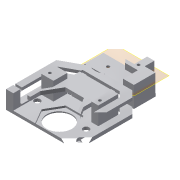
# Autodesk Inventor part: 06_Case_Upper_v1
Saved by Autodesk Inventor 2016 (Build 200138000, 138)
## iProperties
Created: 2017-11-17
Part Number: 06_Case_Upper_v1
Material: Generisch
Document SubType Name: Modeling
Designer: diederichbenedict
Density: 1 g/cm^3
Appearance: Weiß
Author: diederichbenedict
Autodesk Inventor part; units mm, degrees
ref_plane "YZ Plane" through (0, 0, 0) normal (1, 0, 0) x (0, 1, 0)
ref_plane "XZ Plane" through (0, 0, 0) normal (0, 1, 0) x (-1, 0, 0)
ref_plane "XY Plane" through (0, 0, 0) normal (0, 0, 1) x (1, 0, 0)
ref_plane "Arbeitsebene1" through (-53, 10.5, 0) normal (0, 0, 1) x (1, 0, 0)
sketch "Skizze1" plane through (-53, 10.5, 0) normal (0, 0, 1) x (1, 0, 0)
  circle A0 centre (53, -7.5) radius 1.75 construction
  line L0 (49, 8.5) -> (49, -12.5) construction
  line L1 (49, -12.5) -> (57, -12.5) construction
  line L2 (57, -12.5) -> (57, 8.5) construction
  line L3 (57, 8.5) -> (49, 8.5) construction
  arc A1 (1.4361, -8.5) -> (-1.4361, -8.5) centre (0, -7.5) ccw construction
  line L4 (1.4361, -8.5) -> (4, -8.5) construction
  line L5 (4, -8.5) -> (4, 8.5) construction
  line L6 (4, 8.5) -> (-4, 8.5) construction
  line L7 (-4, 8.5) -> (-4, -8.5) construction
  line L8 (-4, -8.5) -> (-1.4361, -8.5) construction
  line L9 (74, -106.5) -> (69, -111.5) construction
  line L10 (74, -66.5) -> (74, -106.5) construction
  line L11 (64, -66.5) -> (74, -66.5) construction
  line L12 (64, -70.0238) -> (64, -66.5) construction
  line L13 (71.5194, -70.0238) -> (64, -70.0238) construction
  line L14 (71.5194, -74.0238) -> (71.5194, -70.0238) construction
  line L15 (64, -74.0238) -> (71.5194, -74.0238) construction
  line L16 (64, -111.5) -> (64, -74.0238) construction
  line L17 (69, -111.5) -> (64, -111.5) construction
  circle A2 centre (69, -77.2738) radius 1.75 construction
  circle A3 centre (1, -79.0238) radius 1.75 construction
  line L18 (1, -74.0238) -> (6, -82.684) construction
  line L19 (-1, -74.0238) -> (1, -74.0238) construction
  line L20 (-1, -70.0238) -> (-1, -74.0238) construction
  line L21 (0.3943, -66.5) -> (-1, -70.0238) construction
  line L22 (-4, -66.5) -> (0.3943, -66.5) construction
  line L23 (-4, -106.5) -> (-4, -66.5) construction
  line L24 (1, -111.5) -> (-4, -106.5) construction
  line L25 (6, -111.5) -> (1, -111.5) construction
  line L26 (6, -82.684) -> (6, -111.5) construction
  line L27 (-4, -111.5) -> (-4, 8.5) construction
  line L28 (-4, 8.5) -> (4, 8.5) construction
  line L29 (6, 8.5) -> (4, 8.5) construction
  line L30 (74, -66.5) -> (6, -66.5) construction
  line L31 (74, -111.5) -> (74, -66.5) construction
  circle A4 centre (38.7332, -103.6375) radius 17.5 construction
  circle A5 centre (13, 28.5) radius 1 construction
  circle A6 centre (43, -3.5) radius 1 construction
  circle A7 centre (13, -3.5) radius 1 construction
  circle A8 centre (43, 28.5) radius 1 construction
  circle A9 centre (28, 12.5) radius 18.75 construction
  line L32 (48, -3.5) -> (48, 28.5) construction
  arc A10 (43, -8.5) -> (48, -3.5) centre (43, -3.5) ccw construction
  line L33 (13, -8.5) -> (43, -8.5) construction
  arc A11 (8, -3.5) -> (13, -8.5) centre (13, -3.5) ccw construction
  line L34 (8, 28.5) -> (8, -3.5) construction
  arc A12 (13, 33.5) -> (8, 28.5) centre (13, 28.5) ccw construction
  line L35 (43, 33.5) -> (13, 33.5) construction
  arc A13 (48, 28.5) -> (43, 33.5) centre (43, 28.5) ccw construction
  line L36 (74, -111.5) -> (74, -125) construction
  line L37 (74, -125) -> (-4, -125) construction
  line L38 (-4, -125) -> (-4, -111.5) construction
  circle A14 centre (38.7332, -103.6375) radius 17.5 construction
  line L39 (57, 8.5) -> (49, 8.5) construction
  line L40 (49, 8.5) -> (49, -9.5) construction
  line L41 (49, -12.5) -> (57, -12.5) construction
  line L42 (57, -12.5) -> (57, 8.5) construction
  line L43 (6, -9.5) -> (49, -9.5) construction
  line L44 (57, -12.5) -> (49, -12.5) construction
  line L45 (6, -14.5) -> (57, -14.5) construction
  line L46 (57, -14.5) -> (57, -12.5) construction
  line L47 (6, -66.5) -> (6, -14.5) construction
  line L48 (6, -9.5) -> (6, 8.5) construction
  line L49 (49, -12.5) -> (48, -12.5) construction
  line L50 (-4, 8.5) -> (6, 8.5)
  line L51 (6, 8.5) -> (6, -9.5)
  line L52 (6, -9.5) -> (49, -9.5)
  line L53 (49, -9.5) -> (49, 8.5)
  line L54 (57, 8.5) -> (49, 8.5)
  line L55 (57, 8.5) -> (57, -14.5)
  line L56 (57, -14.5) -> (6, -14.5)
  line L57 (6, -14.5) -> (6, -66.5)
  line L58 (6, -66.5) -> (74, -66.5)
  line L59 (74, -66.5) -> (74, -125)
  line L60 (74, -125) -> (-4, -125)
  line L61 (-4, -125) -> (-4, 8.5)
  circle A15 centre (38.7332, -103.6375) radius 17.5
  circle A16 centre (1, -96.5) radius 4.25
  circle A17 centre (69, -96.5) radius 4.25
  circle A18 centre (0, 3.5) radius 3.5
  circle A19 centre (53, 3.5) radius 3.5
  line L62 (57, 8.5) -> (59, 8.5)
  line L63 (59, 8.5) -> (59, -14.5)
  line L64 (59, -14.5) -> (57, -14.5)
  line L65 (57, -14.5) -> (57, 8.5)
  line L66 (6, -14.5) -> (13, -14.5)
  line L67 (13, -14.5) -> (13, -66.5)
  line L68 (13, -66.5) -> (6, -66.5)
  line L69 (6, -66.5) -> (6, -14.5)
  line L70 (74, -106.5) -> (69, -111.5) projected
  line L71 (74, -66.5) -> (74, -106.5) projected
  line L72 (64, -70.0238) -> (64, -66.5) projected
  line L73 (71.5194, -70.0238) -> (64, -70.0238) projected
  line L74 (71.5194, -74.0238) -> (71.5194, -70.0238) projected
  line L75 (64, -74.0238) -> (71.5194, -74.0238) projected
  line L76 (64, -111.5) -> (64, -74.0238) projected
  line L77 (69, -111.5) -> (64, -111.5) projected
  arc A20 (1.4361, -8.5) -> (1, -8.9361) centre (0, -7.5) ccw projected
  line L78 (1.4361, -8.5) -> (4, -8.5) projected
  line L79 (4, -8.5) -> (4, 8.5) projected
  line L80 (4, 8.5) -> (-4, 8.5) projected
  line L81 (-4, 8.5) -> (-4, -19.0851) projected
  line L82 (49, 8.5) -> (49, -12.5) projected
  line L83 (57, 8.5) -> (49, 8.5) projected
  line L84 (59, -14.5) -> (74, -14.5)
  line L85 (74, -14.5) -> (74, -4.5)
  line L86 (74, -4.5) -> (59, -4.5)
  line L87 (59, -4.5) -> (59, -14.5)
  line L88 (74, -14.5) -> (59, -14.5)
  line L89 (59, -14.5) -> (59, -35)
  line L90 (59, -35) -> (74, -35)
  line L91 (74, -35) -> (74, -14.5)
  line L92 (-4, -19.0851) -> (1, -19.0851) projected
  line L93 (1, -19.0851) -> (1, -8.9361) projected
  circle A21 centre (1, -96.5) radius 3.75 projected
  circle A22 centre (69, -96.5) radius 3.75 projected
  circle A23 centre (0, 3.5) radius 3 projected
  circle A24 centre (53, 3.5) radius 3 projected
  point P0 (53, -10.5)
  dimension "d1" = 2
  dimension "d2" = 8.5
  dimension "d3" = 8.5
  dimension "d4" = 7
  dimension "d5" = 7
  constraints: 95 end point, 21 perpendicular, 13 parallel, 8 horizontal, 8 point on line, 6 centre point, 3 vertical, 2 coincident, 1 collinear, 1 concentric
  measures "d1" distance between parallel lines of L45 L44
  measures "d2" diameter of A16
  measures "d3" diameter of A17
  measures "d4" diameter of A18
  measures "d5" diameter of A19
extrude "Extrusion1" add sketch "Skizze1" along normal blind 4 contours L50 L79 L78 A20 L93 L92 L61 | L50 L51 L52 L53 L54 L55 L56 L57 L58 L72 L73 L74 L75 L76 L77 L70 L59 L60 L61 L92 L93 A20 L78 L79 | L70 L77 L76 L75 L74 L73 L72 L58 L59 | L62 L63 L64 L55 | L58 L57 L56 L67 | L63 L86 L85 L84 | L84 L91 L90 L89
sketch "Skizze2" plane through (-53, 10.5, 4) normal (0, 0, 1) x (1, 0, 0)
  circle A0 centre (38.7332, -103.6375) radius 18 construction
  line L0 (50.5689, -124.1375) -> (62.4046, -103.6375) construction
  line L1 (62.4046, -103.6375) -> (50.5689, -83.1375) construction
  line L2 (50.5689, -83.1375) -> (26.8975, -83.1375) construction
  line L3 (26.8975, -83.1375) -> (15.0619, -103.6375) construction
  line L4 (15.0619, -103.6375) -> (26.8975, -124.1375) construction
  line L5 (26.8975, -124.1375) -> (50.5689, -124.1375) construction
  line L6 (51.0601, -82.2867) -> (63.387, -103.6375)
  line L7 (63.387, -103.6375) -> (51.0601, -124.9883)
  line L8 (51.0601, -124.9883) -> (26.4063, -124.9883)
  line L9 (26.4063, -124.9883) -> (14.0795, -103.6375)
  line L10 (14.0795, -103.6375) -> (26.4063, -82.2867)
  line L11 (26.4063, -82.2867) -> (51.0601, -82.2867)
  point P0 (53, -10.5)
  dimension "d8" = 0.8508
  constraints: 12 end point, 5 other
  measures "d8" distance between parallel lines of L1 L6
extrude "Extrusion2" cut sketch "Skizze2" against normal blind 2.5
sketch "Skizze4" plane through (-53, 10.5, 0) normal (0, 0, -1) x (-1, 0, 0)
  circle A0 centre (-38.7332, -103.6375) radius 17.5 projected
  circle A1 centre (-69, -96.5) radius 4.25 projected
  circle A2 centre (-1, -96.5) radius 4.25 projected
  circle A3 centre (-53, 3.5) radius 3.5 projected
  circle A4 centre (0, 3.5) radius 3.5 projected
  line L0 (-59, 8.5) -> (-49, 8.5) projected
  line L1 (-59, -4.5) -> (-59, 8.5) projected
  line L2 (-13, -14.5) -> (-59, -14.5) projected
  line L3 (-13, -66.5) -> (-13, -14.5) projected
  line L4 (-74, -66.5) -> (-13, -66.5) projected
  line L5 (-74, -125) -> (-74, -66.5) projected
  line L6 (4, -125) -> (-74, -125) projected
  line L7 (4, 8.5) -> (4, -125) projected
  line L8 (-6, 8.5) -> (4, 8.5) projected
  line L9 (-6, -9.5) -> (-6, 8.5) projected
  line L10 (-49, -9.5) -> (-6, -9.5) projected
  line L11 (-49, 8.5) -> (-49, -9.5) projected
  line L12 (4, 8.5) -> (4, -125) projected
  line L13 (4, -125) -> (14, -125)
  line L14 (14, -125) -> (14, -115)
  line L15 (14, -115) -> (4, -115)
  line L16 (4, -115) -> (4, -125)
  line L17 (4, -125) -> (-74, -125) projected
  line L18 (-74, -125) -> (-84, -125)
  line L19 (-84, -125) -> (-84, -115)
  line L20 (-84, -115) -> (-74, -115)
  line L21 (-74, -115) -> (-74, -125)
  line L22 (-61.5243, -52.5) -> (-16, -52.5)
  line L23 (-16, -52.5) -> (-16, -64)
  line L24 (-16, -64) -> (-61.5243, -64)
  line L25 (-61.5243, -64) -> (-61.5243, -52.5)
  line L26 (-61.5243, -52.5) -> (-16, -64) construction
  line L27 (-16, -52.5) -> (-61.5243, -64) construction
  line L28 (-74, -4.5) -> (-59, -4.5) projected
  line L29 (-74, -35) -> (-74, -4.5) projected
  line L30 (-59, -35) -> (-74, -35) projected
  line L31 (-59, -14.5) -> (-59, -35) projected
  point P0 (-53, -10.5)
  point P1 (-38.7621, -58.25)
  dimension "d11" = 10
  dimension "d12" = 10
  dimension "d13" = 10
  dimension "d14" = 10
  constraints: 28 end point, 6 parallel, 3 horizontal, 3 perpendicular, 2 midpoint
  measures "d11" distance of L15.end L14.end
  measures "d12" distance of L14.end L13.end
  measures "d13" distance of L19.end L20.end
  measures "d14" distance of L18.end L19.end
extrude "Extrusion3" add sketch "Skizze4" against normal blind 25 contours L15 L14 L13 L7 | L18 L19 L20 L5 | L22 L23 L24 L25
sketch "Skizze5" plane through (-53, 10.5, 0) normal (0, 0, -1) x (-1, 0, 0)
  circle A0 centre (-38.7332, -103.6375) radius 17.5 projected
  circle A1 centre (-69, -96.5) radius 4.25 projected
  circle A2 centre (-1, -96.5) radius 4.25 projected
  circle A3 centre (-53, 3.5) radius 3.5 projected
  circle A4 centre (0, 3.5) radius 3.5 projected
  line L0 (-59, 8.5) -> (-49, 8.5) projected
  line L1 (-59, -4.5) -> (-59, 8.5) projected
  line L2 (-13, -14.5) -> (-59, -14.5) projected
  line L3 (-13, -66.5) -> (-13, -14.5) projected
  line L4 (-74, -66.5) -> (-13, -66.5) projected
  line L5 (-74, -115) -> (-74, -66.5) projected
  line L6 (-74, -115) -> (-84, -115) projected
  line L7 (-84, -115) -> (-84, -125) projected
  line L8 (-84, -125) -> (14, -125) projected
  line L9 (14, -125) -> (14, -115) projected
  line L10 (14, -115) -> (4, -115) projected
  line L11 (4, 8.5) -> (4, -115) projected
  line L12 (-6, 8.5) -> (4, 8.5) projected
  line L13 (-6, -9.5) -> (-6, 8.5) projected
  line L14 (-49, -9.5) -> (-6, -9.5) projected
  line L15 (-49, 8.5) -> (-49, -9.5) projected
  line L16 (-84, -115) -> (-75, -115)
  line L17 (-75, -115) -> (-75, -66.5)
  line L18 (-75, -66.5) -> (-84, -66.5)
  line L19 (-84, -66.5) -> (-84, -115)
  line L20 (14, -115) -> (5, -115)
  line L21 (5, -115) -> (5, -66.5)
  line L22 (5, -66.5) -> (14, -66.5)
  line L23 (14, -66.5) -> (14, -115)
  line L24 (-75.5, -38.5) -> (-16, -38.5)
  line L25 (-16, -38.5) -> (-16, -48.5)
  line L26 (-16, -48.5) -> (-67.8163, -48.5)
  line L27 (-67.8163, -48.5) -> (-24.5519, -48.5) construction
  line L28 (-75.5, -38.5) -> (-84, -47)
  line L29 (-84, -47) -> (-84, -66.5)
  line L30 (-16, -48.5) -> (9.4471, -48.5) construction
  line L31 (-16, -38.5) -> (27.2951, -38.5) construction
  line L32 (5, -66.5) -> (14, -66.5) construction
  line L33 (14, -66.5) -> (14, -54.9004) construction
  line L34 (14, -54.9004) -> (5, -54.9004) construction
  line L35 (5, -54.9004) -> (5, -66.5) construction
  line L36 (5, -66.5) -> (14, -66.5)
  line L37 (14, -66.5) -> (14, -54.9004)
  line L38 (14, -54.9004) -> (5, -54.9004)
  line L39 (5, -54.9004) -> (5, -66.5)
  line L40 (-82.6105, -46.7432) -> (-47.3709, -46.7432) construction
  line L41 (-67.8163, -48.5) -> (-75, -55.6837)
  line L42 (-67.8163, -48.5) -> (-57.6571, -48.5) construction
  line L43 (-75, -55.6837) -> (-75, -66.5)
  line L44 (-16, -52.5) -> (-16, -64) projected
  line L45 (-61.5243, -52.5) -> (-16, -52.5) projected
  line L46 (-16, -48.5) -> (-22, -48.5)
  line L47 (-22, -48.5) -> (-22, -52.5)
  line L48 (-22, -52.5) -> (-16, -52.5)
  line L49 (-16, -52.5) -> (-16, -48.5)
  line L50 (-61.5243, -52.5) -> (-55.5243, -52.5)
  line L51 (-55.5243, -52.5) -> (-55.5243, -48.5)
  line L52 (-55.5243, -48.5) -> (-61.5243, -48.5)
  line L53 (-61.5243, -48.5) -> (-61.5243, -52.5)
  circle A5 centre (-38.7332, -103.6375) radius 13.419 projected
  line L54 (-36, -18.5) -> (-16, -18.5)
  line L55 (-16, -18.5) -> (-16, -38.5)
  line L56 (-16, -38.5) -> (-36, -38.5)
  line L57 (-36, -38.5) -> (-36, -18.5)
  line L58 (-36, -18.5) -> (-16, -38.5) construction
  line L59 (-16, -18.5) -> (-36, -38.5) construction
  line L60 (-74, -4.5) -> (-59, -4.5) projected
  line L61 (-74, -35) -> (-74, -4.5) projected
  line L62 (-59, -35) -> (-74, -35) projected
  line L63 (-59, -14.5) -> (-59, -35) projected
  point P0 (-53, -10.5)
  point P1 (-26, -28.5)
  dimension "d23" = 135
  dimension "d24" = 135
  dimension "d25" = 1
  dimension "d28" = 10
  dimension "d29" = 4
  dimension "d30" = 6
  dimension "d31" = 4
  dimension "d32" = 6
  dimension "d33" = 10
  dimension "d34" = 10
  constraints: 84 end point, 15 parallel, 13 horizontal, 8 perpendicular, 3 point on line, 2 midpoint, 2 vertical, 1 collinear, 1 equal length
  measures "d23" angle of L29 L28
  measures "d24" angle of L41 L42
  measures "d25" distance between parallel lines of L17 L5
  measures "d28" distance between parallel lines of L24 L27
  measures "d29" distance between parallel lines of L26 L45
  measures "d30" distance of L52.end L51.end
  measures "d31" distance of L51.end L50.end
  measures "d32" distance between parallel lines of L47 L49
  measures "d33" distance from line of L24 point (-26, -28.5)
  measures "d34" distance from line of point (-26, -28.5) L55
extrude "Extrusion4" add sketch "Skizze5" against normal blind 5 contours L21 L22 L23 L10 | L39 L38 L37 L22 | L6 L19 L18 L17 | L18 L29 L28 L24 L25 L26 L41 L43 | L26 L51 L45 L53 | L57 L54 L55 L24 | L26 L49 L45 L47
sketch "Skizze6" plane through (-53, 10.5, 25) normal (0, 0, 1) x (1, 0, 0)
  circle A0 centre (38, -71.483) radius 4.4 construction
  circle A1 centre (38, -21.483) radius 4.4 construction
  circle A2 centre (38, -46.483) radius 4 construction
  line L0 (25, -81.483) -> (51, -81.483) construction
  line L1 (51, -81.483) -> (63.7116, -103.5) construction
  line L2 (63.7116, -103.5) -> (63.7116, -117.5) construction
  line L3 (63.7116, -117.5) -> (67.7116, -117.5) construction
  line L4 (67.7116, -117.5) -> (67.7116, -103.5) construction
  line L5 (67.7116, -103.5) -> (51, -74.5548) construction
  line L6 (51, -74.5548) -> (51, -11.483) construction
  line L7 (51, -11.483) -> (25, -11.483) construction
  line L8 (25, -11.483) -> (25, -74.5549) construction
  line L9 (25, -74.5549) -> (8.2885, -103.5) construction
  line L10 (8.2885, -103.5) -> (8.2885, -117.5) construction
  line L11 (8.2885, -117.5) -> (12.2885, -117.5) construction
  line L12 (12.2885, -117.5) -> (12.2885, -103.5) construction
  line L13 (12.2885, -103.5) -> (25, -81.483) construction
  line L14 (8.2885, -117.5) -> (12.2885, -117.5)
  line L15 (63.7116, -117.5) -> (67.7116, -117.5)
  line L16 (16, -64) -> (61.5243, -64) projected
  line L17 (16, -64) -> (16, -80.0255)
  line L18 (61.5243, -64) -> (61.5243, -81.5137)
  line L19 (8.2885, -117.5) -> (8.2885, -103.5)
  line L20 (16, -80.0255) -> (16, -90.1433)
  line L21 (8.2885, -103.5) -> (16, -90.1433)
  line L22 (12.2885, -117.5) -> (12.2885, -103.5)
  line L23 (12.2885, -103.5) -> (25, -81.483)
  line L24 (25, -81.483) -> (51, -81.483)
  line L25 (51, -81.483) -> (63.7116, -103.5)
  line L26 (63.7116, -103.5) -> (63.7116, -117.5)
  line L27 (67.7116, -117.5) -> (67.7116, -103.5)
  line L28 (67.7116, -103.5) -> (51, -74.5548)
  line L29 (61.5243, -81.5137) -> (61.5243, -92.7834)
  point P0 (53, -10.5)
  constraints: 30 end point, 7 parallel, 2 perpendicular, 2 point on line, 1 horizontal, 1 vertical
extrude "Extrusion5" add sketch "Skizze6" against normal blind 5
sketch "Skizze7" plane through (-53, 10.5, 5) normal (0, 0, 1) x (1, 0, 0)
  line L0 (-5, -115) -> (-5, -54.9004) projected
  line L1 (-5, -54.9004) -> (-14, -54.9004) projected
  line L2 (-14, -54.9004) -> (-14, -115) projected
  line L3 (-5, -115) -> (-14, -115) projected
  line L4 (84, -115) -> (75, -115) projected
  line L5 (84, -115) -> (84, -47) projected
  line L6 (84, -47) -> (75.5, -38.5) projected
  line L7 (75.5, -38.5) -> (36, -38.5) projected
  line L8 (36, -38.5) -> (36, -18.5) projected
  line L9 (36, -18.5) -> (16, -18.5) projected
  line L10 (16, -18.5) -> (16, -52.5) projected
  line L11 (22, -52.5) -> (16, -52.5) projected
  line L12 (22, -52.5) -> (22, -48.5) projected
  line L13 (22, -48.5) -> (55.5243, -48.5) projected
  line L14 (55.5243, -48.5) -> (55.5243, -52.5) projected
  line L15 (61.5243, -52.5) -> (55.5243, -52.5) projected
  line L16 (61.5243, -52.5) -> (61.5243, -48.5) projected
  line L17 (61.5243, -48.5) -> (67.8163, -48.5) projected
  line L18 (67.8163, -48.5) -> (75, -55.6837) projected
  line L19 (75, -55.6837) -> (75, -115) projected
  line L20 (-14, -54.9004) -> (-14, -115) projected
  line L21 (-14, -54.9004) -> (-5, -54.9004)
  line L22 (-5, -54.9004) -> (-5, -61.9004)
  line L23 (-5, -61.9004) -> (-14, -61.9004)
  line L24 (-14, -61.9004) -> (-14, -54.9004)
  line L25 (16, -38.5) -> (28.7408, -38.5)
  line L26 (28.7408, -38.5) -> (28.7408, -48.5)
  line L27 (28.7408, -48.5) -> (16, -48.5)
  line L28 (16, -48.5) -> (16, -38.5)
  point P0 (53, -10.5)
  dimension "d35" = 9
  dimension "d36" = 7
  constraints: 16 end point, 4 parallel, 2 horizontal, 2 perpendicular, 1 point on line
  measures "d35" distance of L22.end L23.end
  measures "d36" distance of L21.end L22.end
extrude "Extrusion6" add sketch "Skizze7" along normal blind 3 contours L23 L2 L1 L0 | L25 L26 L13 L27 L10
sketch "Skizze8" plane through (-53, 10.5, 8) normal (0, 0, 1) x (1, 0, 0)
  line L0 (-14, -54.9004) -> (-14, -61.9004) projected
  line L1 (-14, -61.9004) -> (-5, -61.9004) projected
  line L2 (-5, -61.9004) -> (-5, -54.9004) projected
  line L3 (-5, -54.9004) -> (-14, -54.9004) projected
  line L4 (16, -38.5) -> (16, -48.5) projected
  line L5 (16, -48.5) -> (28.7408, -48.5) projected
  line L6 (28.7408, -48.5) -> (28.7408, -38.5) projected
  line L7 (28.7408, -38.5) -> (16, -38.5) projected
  line L8 (-14, -54.9004) -> (16, -38.5)
  line L9 (-5, -61.9004) -> (19.5123, -48.5)
  point P0 (53, -10.5)
  constraints: 4 end point, 1 parallel, 1 point on line
extrude "Extrusion7" add sketch "Skizze8" along normal blind 3
sketch "Skizze9" plane through (-53, 10.5, 25) normal (0, 0, 1) x (1, 0, 0)
  line L0 (74, -115) -> (74, -125) projected
  line L1 (74, -125) -> (84, -125) projected
  line L2 (84, -125) -> (84, -115) projected
  line L3 (84, -115) -> (74, -115) projected
  line L4 (-14, -125) -> (-4, -125) projected
  line L5 (-4, -125) -> (-4, -115) projected
  line L6 (-4, -115) -> (-14, -115) projected
  line L7 (-14, -115) -> (-14, -125) projected
  line L8 (-5, -61.9004) -> (-14, -61.9004) projected
  line L9 (-14, -61.9004) -> (-14, -115) projected
  line L10 (-5, -115) -> (-14, -115) projected
  line L11 (-5, -115) -> (-5, -61.9004) projected
  line L12 (-14, -54.9004) -> (-14, -61.9004) projected
  line L13 (-14, -61.9004) -> (-5, -61.9004) projected
  line L14 (-5, -61.9004) -> (19.5123, -48.5) projected
  line L15 (19.5123, -48.5) -> (28.7408, -48.5) projected
  line L16 (28.7408, -48.5) -> (28.7408, -38.5) projected
  line L17 (28.7408, -38.5) -> (16, -38.5) projected
  line L18 (16, -38.5) -> (-14, -54.9004) projected
  line L19 (28.7408, -38.5) -> (28.7408, -48.5) projected
  line L20 (28.7408, -48.5) -> (55.5243, -48.5) projected
  line L21 (55.5243, -48.5) -> (55.5243, -52.5) projected
  line L22 (61.5243, -52.5) -> (55.5243, -52.5) projected
  line L23 (61.5243, -52.5) -> (61.5243, -48.5) projected
  line L24 (61.5243, -48.5) -> (67.8163, -48.5) projected
  line L25 (67.8163, -48.5) -> (75, -55.6837) projected
  line L26 (75, -55.6837) -> (75, -115) projected
  line L27 (84, -115) -> (75, -115) projected
  line L28 (84, -115) -> (84, -47) projected
  line L29 (84, -47) -> (75.5, -38.5) projected
  line L30 (75.5, -38.5) -> (36, -38.5) projected
  line L31 (36, -38.5) -> (36, -18.5) projected
  line L32 (36, -18.5) -> (16, -18.5) projected
  line L33 (36, -38.5) -> (16, -38.5)
  line L34 (22, -48.5) -> (16, -48.5) projected
  line L35 (16, -48.5) -> (16, -52.5) projected
  line L36 (22, -52.5) -> (16, -52.5) projected
  line L37 (22, -52.5) -> (22, -48.5) projected
  line L38 (16, -18.5) -> (16, -38.5) projected
  line L39 (16, -38.5) -> (28.7408, -38.5) projected
  point P0 (53, -10.5)
  constraints: 2 end point, 1 horizontal
extrude "Extrusion8" add sketch "Skizze9" against normal blind 4
sketch "Skizze10" plane through (-53, 10.5, 5) normal (0, 0, 1) x (1, 0, 0)
  line L0 (-5, -61.9004) -> (-14, -61.9004) projected
  line L1 (-14, -61.9004) -> (-14, -115) projected
  line L2 (-5, -115) -> (-14, -115) projected
  line L3 (-5, -115) -> (-5, -61.9004) projected
  line L4 (28.7408, -38.5) -> (28.7408, -48.5) projected
  line L5 (28.7408, -48.5) -> (55.5243, -48.5) projected
  line L6 (55.5243, -48.5) -> (55.5243, -52.5) projected
  line L7 (61.5243, -52.5) -> (55.5243, -52.5) projected
  line L8 (61.5243, -52.5) -> (61.5243, -48.5) projected
  line L9 (61.5243, -48.5) -> (67.8163, -48.5) projected
  line L10 (67.8163, -48.5) -> (75, -55.6837) projected
  line L11 (75, -55.6837) -> (75, -115) projected
  line L12 (84, -115) -> (75, -115) projected
  line L13 (84, -115) -> (84, -47) projected
  line L14 (84, -47) -> (75.5, -38.5) projected
  line L15 (75.5, -38.5) -> (36, -38.5) projected
  line L16 (36, -38.5) -> (36, -18.5) projected
  line L17 (36, -18.5) -> (16, -18.5) projected
  line L18 (84, -115) -> (84, -47) projected
  line L19 (84, -115) -> (75, -115)
  line L20 (75, -115) -> (75, -112)
  line L21 (75, -112) -> (84, -112)
  line L22 (84, -112) -> (84, -115)
  line L23 (-14, -115) -> (-5, -115)
  line L24 (-5, -115) -> (-5, -112)
  line L25 (-5, -112) -> (-14, -112)
  line L26 (-14, -112) -> (-14, -115)
  line L27 (67.8163, -48.5) -> (61.5243, -48.5) projected
  line L28 (61.5243, -48.5) -> (55.5243, -48.5)
  line L29 (55.5243, -48.5) -> (55.5243, -52.5)
  line L30 (55.5243, -52.5) -> (61.5243, -52.5)
  line L31 (61.5243, -52.5) -> (61.5243, -48.5)
  line L32 (22, -52.5) -> (16, -52.5) projected
  line L33 (22, -52.5) -> (16, -52.5)
  line L34 (16, -52.5) -> (16, -48.5)
  line L35 (16, -48.5) -> (22, -48.5)
  line L36 (22, -48.5) -> (22, -52.5)
  line L37 (16, -18.5) -> (16, -38.5) projected
  line L38 (16, -38.5) -> (28.7408, -38.5) projected
  point P0 (53, -10.5)
  constraints: 32 end point, 8 parallel, 4 horizontal, 4 perpendicular, 4 point on line
extrude "Extrusion9" cut sketch "Skizze10" against normal blind 4.3 contours L3 L2 L1 L25 | L28 L8 L7 L6 | L21 L13 L12 L11 | L32 L34 L35 L36
sketch "Skizze11" plane through (-53, 10.5, 25) normal (0, 0, 1) x (1, 0, 0)
  line L0 (22, -52.5) -> (22, -48.5) projected
  line L1 (55.5243, -48.5) -> (22, -48.5) projected
  line L2 (55.5243, -52.5) -> (55.5243, -48.5) projected
  line L3 (55.5243, -52.5) -> (22, -52.5) projected
  line L4 (-14, -125) -> (-4, -125) projected
  line L5 (-4, -125) -> (-4, -115) projected
  line L6 (-4, -115) -> (-5, -115) projected
  line L7 (-5, -115) -> (-5, -61.9004) projected
  line L8 (-5, -61.9004) -> (16, -50.4201) projected
  line L9 (16, -50.4201) -> (16, -90.1433) projected
  line L10 (61.5243, -48.5) -> (61.5243, -81.5137) projected
  line L11 (67.8163, -48.5) -> (61.5243, -48.5) projected
  line L12 (75, -55.6837) -> (67.8163, -48.5) projected
  line L13 (75, -115) -> (75, -55.6837) projected
  line L14 (75, -115) -> (74, -115) projected
  line L15 (74, -115) -> (74, -125) projected
  line L16 (74, -125) -> (84, -125) projected
  line L17 (84, -125) -> (84, -47) projected
  line L18 (75.5, -38.5) -> (84, -47) projected
  line L19 (16, -38.5) -> (-14, -54.9004) projected
  line L20 (-14, -54.9004) -> (-14, -125) projected
  line L21 (75, -115) -> (75, -112) projected
  line L22 (84, -115) -> (75, -115) projected
  line L23 (84, -112) -> (84, -115) projected
  line L24 (75, -112) -> (84, -112) projected
  line L25 (-5, -115) -> (-14, -115) projected
  line L26 (-5, -112) -> (-5, -115) projected
  line L27 (-14, -112) -> (-5, -112) projected
  line L28 (-14, -115) -> (-14, -112) projected
  line L29 (22, -52.5) -> (16, -52.5) projected
  line L30 (22, -48.5) -> (22, -52.5) projected
  line L31 (16, -48.5) -> (22, -48.5) projected
  line L32 (16, -52.5) -> (16, -48.5) projected
  line L33 (61.5243, -52.5) -> (55.5243, -52.5) projected
  line L34 (61.5243, -48.5) -> (61.5243, -52.5) projected
  line L35 (55.5243, -48.5) -> (61.5243, -48.5) projected
  line L36 (55.5243, -52.5) -> (55.5243, -48.5) projected
  line L37 (8.2885, -103.5) -> (16, -90.1433) projected
  line L38 (8.2885, -117.5) -> (8.2885, -103.5) projected
  line L39 (12.2885, -117.5) -> (8.2885, -117.5) projected
  line L40 (12.2885, -103.5) -> (12.2885, -117.5) projected
  line L41 (25, -81.483) -> (12.2885, -103.5) projected
  line L42 (51, -81.483) -> (25, -81.483) projected
  line L43 (63.7116, -103.5) -> (51, -81.483) projected
  line L44 (63.7116, -117.5) -> (63.7116, -103.5) projected
  line L45 (67.7116, -117.5) -> (63.7116, -117.5) projected
  line L46 (67.7116, -103.5) -> (67.7116, -117.5) projected
  line L47 (61.5243, -92.7834) -> (67.7116, -103.5) projected
  line L48 (61.5243, -81.5137) -> (61.5243, -92.7834) projected
  line L49 (36, -38.5) -> (75.5, -38.5) projected
  line L50 (36, -18.5) -> (36, -38.5) projected
  line L51 (16, -18.5) -> (36, -18.5) projected
  line L52 (16, -38.5) -> (16, -18.5) projected
  point P0 (53, -10.5)
extrude "Extrusion10" cut sketch "Skizze11" against normal blind 3.3 contours L29 L9 L32 L31 L0 | L2 L35 L10 L33 | L7 L25 L20 L27 | L24 L17 L22 L13
sketch "Skizze12" plane through (-53, 10.5, 0) normal (0, 0, -1) x (-1, 0, 0)
  line L0 (-55.5243, -52.5) -> (-55.5243, -48.5) construction
  line L1 (-55.5243, -48.5) -> (-22, -48.5) construction
  line L2 (-22, -48.5) -> (-22, -52.5) construction
  line L3 (-55.5243, -52.5) -> (-22, -52.5) construction
  circle A0 centre (-38.7332, -103.6375) radius 17.5 construction
  circle A1 centre (-69, -96.5) radius 4.25 construction
  circle A2 centre (-1, -96.5) radius 4.25 construction
  circle A3 centre (-53, 3.5) radius 3.5 construction
  circle A4 centre (0, 3.5) radius 3.5 construction
  line L4 (-59, 8.5) -> (-49, 8.5) construction
  line L5 (-59, -4.5) -> (-59, 8.5) construction
  line L6 (-13, -14.5) -> (-59, -14.5) construction
  line L7 (-13, -66.5) -> (-13, -14.5) construction
  line L8 (-74, -66.5) -> (-13, -66.5) construction
  line L9 (-74, -115) -> (-74, -66.5) construction
  line L10 (-74, -115) -> (-75, -115) construction
  line L11 (-75, -115) -> (-75, -55.6837) construction
  line L12 (-75, -55.6837) -> (-67.8163, -48.5) construction
  line L13 (-67.8163, -48.5) -> (-61.5243, -48.5) construction
  line L14 (-61.5243, -64) -> (-61.5243, -48.5) construction
  line L15 (-16, -64) -> (-61.5243, -64) construction
  line L16 (-16, -64) -> (-16, -18.5) construction
  line L17 (-36, -38.5) -> (-75.5, -38.5) construction
  line L18 (-16, -18.5) -> (-36, -18.5) construction
  line L19 (-36, -18.5) -> (-36, -38.5) construction
  line L20 (-75.5, -38.5) -> (-84, -47) construction
  line L21 (-84, -47) -> (-84, -125) construction
  line L22 (-84, -125) -> (14, -125) construction
  line L23 (14, -125) -> (14, -54.9004) construction
  line L24 (14, -54.9004) -> (5, -54.9004) construction
  line L25 (5, -54.9004) -> (5, -115) construction
  line L26 (5, -115) -> (4, -115) construction
  line L27 (4, 8.5) -> (4, -115) construction
  line L28 (-6, 8.5) -> (4, 8.5) construction
  line L29 (-6, -9.5) -> (-6, 8.5) construction
  line L30 (-49, -9.5) -> (-6, -9.5) construction
  line L31 (-49, 8.5) -> (-49, -9.5) construction
  line L32 (-74, -66.5) -> (-13, -66.5) projected
  line L33 (-74, -66.5) -> (-64, -66.5)
  line L34 (-64, -66.5) -> (-64, -56.5)
  line L35 (-64, -56.5) -> (-74, -56.5)
  line L36 (-74, -56.5) -> (-74, -66.5)
  line L37 (-74, -66.5) -> (-64, -66.5)
  line L38 (-64, -66.5) -> (-64, -84.5)
  line L39 (-64, -84.5) -> (-74, -84.5)
  line L40 (-74, -84.5) -> (-74, -66.5)
  circle A5 centre (-69, -77.2738) radius 5 projected
  circle A6 centre (-1, -79.0238) radius 5 projected
  circle A7 centre (-53, 3.5) radius 5 projected
  line L41 (-61.5243, -64) -> (-61.5243, -81.5137) projected
  line L42 (-13, -66.5) -> (4, -66.5)
  line L43 (4, -66.5) -> (4, -86)
  line L44 (4, -86) -> (-13, -86)
  line L45 (-13, -86) -> (-13, -66.5)
  line L46 (-74, -4.5) -> (-59, -4.5) projected
  line L47 (-74, -35) -> (-74, -4.5) projected
  line L48 (-59, -35) -> (-74, -35) projected
  line L49 (-59, -14.5) -> (-59, -35) projected
  point P0 (-53, -10.5)
  dimension "d47" = 10
  dimension "d48" = 10
  dimension "d49" = 10
  dimension "d50" = 18
  constraints: 24 end point, 6 parallel, 3 horizontal, 3 perpendicular, 1 point on line
  measures "d47" distance of L35.end L34.end
  measures "d48" distance of L34.end L33.end
  measures "d49" distance of L38.end L39.end
  measures "d50" distance of L37.end L38.end
ref_plane "Arbeitsebene2" through (-57, -73.6285, 29) normal (0, 0, -1) x (0, 1, 0)
extrude "Extrusion11" add sketch "Skizze12" against normal up to surface (29 mm away) contours L36 L35 L34 L32 | L32 L38 A5 L40 | A5 L38 L39 L40 | A5 | A6 | L43 L44 L45 L42
sketch "Skizze13" plane through (-53, 10.5, 4) normal (0, 0, 1) x (1, 0, 0)
  line L0 (6, -9.5) -> (6, 8.5) projected
  line L1 (6, -9.5) -> (13, -9.5)
  line L2 (13, -9.5) -> (13, -36)
  line L3 (13, -36) -> (6, -36)
  line L4 (6, -36) -> (6, -9.5)
  line L5 (13, -14.5) -> (49, -14.5)
  line L6 (49, -14.5) -> (49, -9.5)
  line L7 (49, -9.5) -> (13, -9.5)
  line L8 (13, -9.5) -> (13, -14.5)
  line L9 (49, 8.5) -> (59, 8.5)
  line L10 (59, 8.5) -> (59, -14.5)
  line L11 (59, -14.5) -> (49, -14.5)
  line L12 (49, -14.5) -> (49, 8.5)
  line L13 (59, -5) -> (74, -5)
  line L14 (74, -5) -> (74, -35)
  line L15 (74, -35) -> (59, -35)
  line L16 (59, -35) -> (59, -5)
  point P0 (53, -10.5)
  constraints: 32 end point, 8 parallel, 4 horizontal, 4 perpendicular, 4 point on line
extrude "Extrusion12" add sketch "Skizze13" along normal up to surface (25 mm away)
ref_plane "Arbeitsebene3" through (-40, -4, 19) normal (0, 0, 1) x (1, 0, 0)
sketch "Skizze14" plane through (-40, -4, 19) normal (0, 0, 1) x (1, 0, 0)
  line L0 (0, 0) -> (46, 0)
  line L1 (46, 0) -> (46, -21)
  line L2 (46, -21) -> (0, -21)
  line L3 (0, -21) -> (0, 0)
  point P0 (40, 4)
  constraints: 8 end point, 2 parallel, 1 horizontal, 1 perpendicular
extrude "Extrusion13" add sketch "Skizze14" along normal blind 2
sketch "Skizze15" plane through (-53, 10.5, 0) normal (0, 0, -1) x (-1, 0, 0)
  circle A0 centre (-1, -96.5) radius 4.25 projected
  circle A1 centre (-69, -96.5) radius 4.25 projected
  circle A2 centre (-38.7332, -103.6375) radius 17.5 projected
  line L0 (-55.5243, -52.5) -> (-55.5243, -48.5) projected
  line L1 (-55.5243, -48.5) -> (-22, -48.5) projected
  line L2 (-22, -48.5) -> (-22, -52.5) projected
  line L3 (-55.5243, -52.5) -> (-22, -52.5) projected
  line L4 (4, 8.5) -> (4, -115) projected
  line L5 (-6, 8.5) -> (4, 8.5) projected
  line L6 (-6, -9.5) -> (-6, 8.5) projected
  line L7 (-49, -9.5) -> (-6, -9.5) projected
  line L8 (-49, 8.5) -> (-49, -9.5) projected
  line L9 (-59, 8.5) -> (-49, 8.5) projected
  line L10 (-59, -4.5) -> (-59, 8.5) projected
  line L11 (-74, -4.5) -> (-59, -4.5) projected
  line L12 (-74, -35) -> (-74, -4.5) projected
  line L13 (-59, -35) -> (-74, -35) projected
  line L14 (-59, -14.5) -> (-59, -35) projected
  line L15 (-13, -14.5) -> (-59, -14.5) projected
  line L16 (-13, -66.5) -> (-13, -14.5) projected
  line L17 (-64, -66.5) -> (-13, -66.5) projected
  line L18 (-64, -66.5) -> (-64, -56.5) projected
  line L19 (-64, -56.5) -> (-74, -56.5) projected
  line L20 (-74, -115) -> (-74, -56.5) projected
  line L21 (-74, -115) -> (-75, -115) projected
  line L22 (-75, -115) -> (-75, -55.6837) projected
  line L23 (-75, -55.6837) -> (-67.8163, -48.5) projected
  line L24 (-67.8163, -48.5) -> (-61.5243, -48.5) projected
  line L25 (-61.5243, -64) -> (-61.5243, -48.5) projected
  line L26 (-16, -64) -> (-61.5243, -64) projected
  line L27 (-16, -64) -> (-16, -18.5) projected
  line L28 (-36, -38.5) -> (-75.5, -38.5) projected
  line L29 (-16, -18.5) -> (-36, -18.5) projected
  line L30 (-36, -18.5) -> (-36, -38.5) projected
  line L31 (-75.5, -38.5) -> (-84, -47) projected
  line L32 (-84, -47) -> (-84, -125) projected
  line L33 (-84, -125) -> (14, -125) projected
  line L34 (14, -125) -> (14, -54.9004) projected
  line L35 (14, -54.9004) -> (5, -54.9004) projected
  line L36 (5, -54.9004) -> (5, -115) projected
  line L37 (5, -115) -> (4, -115) projected
  circle A3 centre (-53, 3.5) radius 3.5 projected
  circle A4 centre (0, 3.5) radius 3.5 projected
  line L38 (-36, -18.5) -> (-16, -18.5)
  line L39 (-16, -18.5) -> (-16, -35)
  line L40 (-16, -35) -> (-36, -35)
  line L41 (-36, -35) -> (-36, -18.5)
  circle A5 centre (-26, -23) radius 2.25
  point P0 (-53, -10.5)
  dimension "d58" = 4.5
  constraints: 8 end point, 2 parallel, 1 centre point, 1 horizontal, 1 perpendicular
  measures "d58" diameter of A5
extrude "Extrusion14" cut sketch "Skizze15" against normal through all contours A5
sketch "Skizze16" plane through (-53, 10.5, 0) normal (0, 0, -1) x (-1, 0, 0)
  circle A0 centre (-26, -23) radius 2.25 projected
  line L0 (-24.33, -25.9689) -> (-27.7361, -25.9307)
  line L1 (-27.7361, -25.9307) -> (-29.4062, -22.9618)
  line L2 (-29.4062, -22.9618) -> (-27.67, -20.0311)
  line L3 (-27.67, -20.0311) -> (-24.2639, -20.0693)
  line L4 (-24.2639, -20.0693) -> (-22.5938, -23.0382)
  line L5 (-22.5938, -23.0382) -> (-24.33, -25.9689)
  point P0 (-53, -10.5)
  dimension "d61" = 5.9
  constraints: 12 end point, 1 coincident, 13 other
  measures "d61" distance between parallel lines of L4 L1
extrude "Extrusion15" cut sketch "Skizze16" against normal blind 4 contours A0 | L0 L1 L2 L3 L4 L5
sketch "Skizze17" plane through (-17, -28, 0) normal (1, 0, 0) x (0, 0, -1)
  line L0 (0, 20) -> (0, 0) projected
  line L1 (0, 20) -> (-5, 20) projected
  line L2 (-5, 0) -> (-5, 20) projected
  line L3 (0, 0) -> (-5, 0) projected
  line L4 (-0.6, 0) -> (-0.6, 2.5)
  line L5 (-0.6, 2.5) -> (-5, 8)
  point P0 (0, 28)
  dimension "d81" = 0.6
  constraints: 4 end point, 2 point on line, 1 vertical
  measures "d81" distance between parallel lines of L0 L4
extrude "Extrusion16" cut sketch "Skizze17" against normal up to surface (20 mm away) contours L3 L2 L5 L4
sketch "Skizze18" plane through (-40, -4, 21) normal (0, 0, 1) x (1, 0, 0)
  circle A0 centre (13, -9) radius 17.5
  line L0 (0, -21.5) -> (0, 0) projected
  line L1 (0, 0) -> (46, 0) projected
  line L2 (46, 0) -> (46, -20.5) projected
  line L3 (46, -20.5) -> (61, -20.5) projected
  line L4 (61, -20.5) -> (61, 9.5) projected
  line L5 (61, 9.5) -> (46, 9.5) projected
  line L6 (46, 9.5) -> (46, 23) projected
  line L7 (46, 23) -> (36, 23) projected
  line L8 (36, 23) -> (36, 5) projected
  line L9 (36, 5) -> (-7, 5) projected
  line L10 (-7, 5) -> (-7, -21.5) projected
  line L11 (-7, -21.5) -> (0, -21.5) projected
  line L12 (36, 5) -> (-7, 5) projected
  line L13 (0, 0) -> (0, -21) projected
  line L14 (-9, 9.5) -> (3, 9.5)
  line L15 (3, 9.5) -> (3, -23.3614)
  line L16 (3, -23.3614) -> (-9, -23.3614)
  line L17 (-9, -23.3614) -> (-9, 9.5)
  point P0 (2.5, 5)
  constraints: 8 end point, 2 parallel, 2 point on circle, 1 centre point, 1 coincident, 1 horizontal, 1 perpendicular, 1 point on line
extrude "Extrusion17" cut sketch "Skizze18" along normal through all contours L15 L1 A0 | L16 L17 L14 L15 A0 L9 L10 L11 L0 | A0 L0 L1 L15 | L0 L11 L10 L9 A0 | A0 L9 L15 L1 L0 | L15 L9 A0 L1 | A0 L15 L9 | L15 A0 L9
sketch "Skizze19" plane through (6, -24.5, 29) normal (0, 0, 1) x (1, 0, 0)
  arc A0 (-57.5639, 26.5) -> (-58, 26.0639) centre (-59, 27.5) ccw projected
  circle A1 centre (-6, 27.5) radius 1.75 projected
  circle A2 centre (-58, -44.0238) radius 1.75 projected
  circle A3 centre (10, -42.2738) radius 1.75 projected
  point P0 (-6, 24.5)
hole "Bohrung1" at (0, 3, 29) at (-53, 3, 29) at (-52, -68.5238, 29) at (16, -66.7738, 29) direction (0, 0, -1) diameter 4 end through all
chamfer "Fase1" distance 5 angle 45 8 edges at (21, 5.5, 16.5) (21, 6, 2) (6, 5.5, 16.5) (-4, 1, 14.5) (-47, 1, 12.5) (-47, -25.5, 12.5) (21, -24.5, 16.5) (21, -24.5, 2)
chamfer "Fase2" distance 10 angle 45 1 edges at (6, -14.25, 19)
